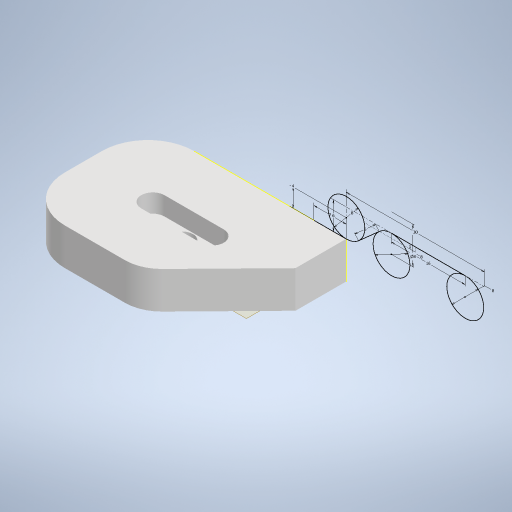
# Autodesk Inventor part: klesce_baza
Saved by Autodesk Inventor 2024 (Build 280153000, 153)
## iProperties
Created: 2023-09-10
Part Number: klesce_baza
Material: Generic
Document SubType Name: Modeling
Designer: jebes windows
Density: 1 g/cm^3
Appearance: Default
Author: jebes windows
Autodesk Inventor part; units mm, degrees
ref_plane "YZ Plane" through (0, 0, 0) normal (1, 0, 0) x (0, 1, 0)
ref_plane "XZ Plane" through (0, 0, 0) normal (0, 1, 0) x (-1, 0, 0)
ref_plane "XY Plane" through (0, 0, 0) normal (0, 0, 1) x (1, 0, 0)
ref_plane "Work Plane1" through (0, 0, 0) normal (0, 0, 1) x (1, 0, 0)
sketch "Sketch1" plane through (0, 0, 0) normal (0, 0, 1) x (1, 0, 0)
  line L0 (14.1591, 1.997) -> (2.2091, 2.65) projected
  arc A0 (2.2091, 2.65) -> (-2.2091, 2.65) centre (0, 0) ccw projected
  line L1 (-2.2091, 2.65) -> (-14.1591, 1.997) projected
  arc A1 (-14.1591, 1.997) -> (-14.1591, -1.997) centre (-14.05, 0) ccw projected
  line L2 (-14.1591, -1.997) -> (-2.2091, -2.65) projected
  arc A2 (-2.2091, -2.65) -> (2.2091, -2.65) centre (0, 0) ccw projected
  line L3 (2.2091, -2.65) -> (14.1591, -1.997) projected
  arc A3 (14.1591, -1.997) -> (14.1591, 1.997) centre (14.05, 0) ccw projected
  circle A4 centre (12.45, 0) radius 0.6 projected
  circle A5 centre (14.45, 0) radius 0.6 projected
  circle A6 centre (10.45, 0) radius 0.6 projected
  circle A7 centre (8.45, 0) radius 0.6 projected
  circle A8 centre (6.45, 0) radius 0.6 projected
  circle A9 centre (4.45, 0) radius 0.6 projected
  circle A10 centre (0, 0) radius 2.3 projected
  circle A11 centre (-4.45, 0) radius 0.6 projected
  circle A12 centre (-6.45, 0) radius 0.6 projected
  circle A13 centre (-8.45, 0) radius 0.6 projected
  circle A14 centre (-10.45, 0) radius 0.6 projected
  circle A15 centre (-12.45, 0) radius 0.6 projected
  circle A16 centre (-14.45, 0) radius 0.6 projected
  line L4 (-21.5, 14) -> (21.5, 14)
  line L5 (21.5, 14) -> (21.5, -14)
  line L6 (21.5, -14) -> (-21.5, -14)
  line L7 (-21.5, -14) -> (-21.5, 14)
  line L8 (-21.5, 14) -> (21.5, -14) construction
  line L9 (21.5, 14) -> (-21.5, -14) construction
  point P0 (0, 0)
  dimension "d0" = 43
  dimension "d1" = 28
  constraints: 12 end point, 2 midpoint, 2 parallel, 1 horizontal, 1 perpendicular
  measures "d0" distance of L5.end L6.end
  measures "d1" distance of L4.end L5.end
extrude "Extrusion1" add sketch "Sketch1" along normal blind 8 contours A3 L3 A2 L2 A1 L1 A0 L0 | A4 | A5 | A6 | A7 | A13 | A14 | A15 | A16 | L4 L5 L6 L7
sketch "Sketch2" plane through (0, 0, 8) normal (0, 0, 1) x (1, 0, 0)
  circle A0 centre (6.45, 0) radius 0.6 projected
  circle A1 centre (6.45, 0) radius 2.5
  circle A2 centre (-6.45, 0) radius 0.6 projected
  circle A3 centre (-6.45, 0) radius 2.5
  line L0 (-6.45, 2.5) -> (6.45, 2.5)
  line L1 (-6.45, -2.5) -> (6.45, -2.5)
  point P0 (0, 0)
  dimension "d4" = 5
  dimension "d5" = 5
  constraints: 4 end point, 4 point on circle, 2 centre point, 2 coincident, 2 horizontal, 2 tangent
  measures "d4" diameter of A1
  measures "d5" diameter of A3
extrude "Extrusion2" cut sketch "Sketch2" against normal blind 4 contours A1 | A1 L1 A3 L0 | A3 | A2
fillet "Fillet1" radius 10 2 edges at (-21.5, -14, 4) (-21.5, 14, 4)
sketch "Sketch3" plane through (0, 0, 8) normal (0, 0, 1) x (1, 0, 0)
  line L0 (-21.5, -14) -> (1.5, -14)
  line L1 (-11.5, -14) -> (21.5, -14) projected
  circle A0 centre (1.5, -6) radius 8
  line L2 (-21.5, 4) -> (-21.5, -4) projected
  line L3 (21.5, -14) -> (21.5, 14) projected
  line L4 (21.5, 14) -> (21.5, 3)
  line L5 (21.5, 3) -> (7.2178, -11.5952)
  arc A1 (-6.45, 2.5) -> (-6.45, -2.5) centre (-6.45, 0) ccw projected
  line L6 (-6.45, 2.5) -> (6.45, 2.5) projected
  arc A2 (6.45, -2.5) -> (6.45, 2.5) centre (6.45, 0) ccw projected
  line L7 (6.45, -2.5) -> (-6.45, -2.5) projected
  arc A3 (-11.5, 14) -> (-21.5, 4) centre (-11.5, 4) ccw projected
  line L8 (-21.5, 4) -> (-21.5, -4) projected
  arc A4 (-21.5, -4) -> (-11.5, -14) centre (-11.5, -4) ccw projected
  line L9 (-11.5, -14) -> (21.5, -14) projected
  line L10 (21.5, -14) -> (21.5, 14) projected
  line L11 (21.5, 14) -> (-11.5, 14) projected
  point P0 (0, 0)
  dimension "d9" = 23
  dimension "d10" = 16
  dimension "d11" = 90
  dimension "d12" = 0
  dimension "d13" = 8
  dimension "d14" = 11
  constraints: 6 end point, 2 point on circle, 2 point on line, 1 centre point, 1 tangent
  measures "d9" distance of L0.start L0.end
  measures "d10" diameter of A0
  measures "d11" angle of L2 L0
  measures "d12" distance from line of L2 L0.start
  measures "d13" distance from line of L0 A0.centre
  measures "d14" distance of L4.end L3.end
extrude "Extrusion3" cut sketch "Sketch3" against normal through all contours A0 L5 L3 L1
sketch "Sketch4" plane through (21.5, 14, 8) normal (0, 1, 0) x (1, 0, 0)
  line L0 (0, 8) -> (0, 0) projected
  line L1 (0, 0) -> (-7, 0)
  line L2 (0, 0) -> (-33, 0) projected
  circle A0 centre (0, -4) radius 4
  line L3 (0, 0) -> (0, -6) construction
  line L4 (0, -6) -> (30, -6) construction
  line L5 (15, -6) -> (15, -5) construction
  line L6 (15, -5) -> (3.873, -5) construction
  line L7 (2.6589, -1.0116) -> (7.1414, -5)
  circle A1 centre (9.7872, -2) radius 4
  line L8 (9.7872, -6) -> (25.7872, -6)
  circle A2 centre (25.7872, -2) radius 4
  point P0 (-21.5, 8)
  dimension "d25" = 8
  dimension "d28" = 8
  dimension "d17" = 7
  dimension "d18" = 8
  dimension "d19" = 4
  dimension "d20" = 6
  dimension "d21" = 30
  dimension "d23" = 1
  dimension "d24" = 6
  dimension "d26" = 8
  dimension "d27" = 16
  constraints: 14 end point, 4 point on line, 3 point on circle, 2 perpendicular, 2 vertical, 2 vertical alignment, 1 centre point, 1 horizontal, 1 midpoint, 1 tangent, 5 other
  measures "d17" distance of L0.end L1.end
  measures "d18" diameter of A0
  measures "d19" distance from line of L1 A0.centre
  measures "d20" distance of L0.end L3.end
  measures "d21" distance of L3.end L4.end
  measures "d23" distance of L5.start L5.end
  measures "d24" distance of L7.start L7.end
  measures "d26" diameter of point (9.787, -2) L4
  measures "d27" distance of L8.start L8.end
body "Solid1"
